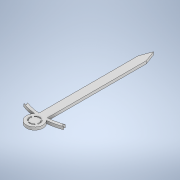
# Autodesk Inventor part: клинок
Saved by Autodesk Inventor 2022 (Build 260153000, 153)
## iProperties
Created: 2023-03-03
Part Number: клинок
Material: Типовые
Document SubType Name: Modeling
Designer: Папа
Density: 1 g/cm^3
Appearance: По умолчанию
Author: Папа
Autodesk Inventor part; units mm, degrees
ref_plane "YZ Plane" through (0, 0, 0) normal (1, 0, 0) x (0, 1, 0)
ref_plane "XZ Plane" through (0, 0, 0) normal (0, 1, 0) x (-1, 0, 0)
ref_plane "XY Plane" through (0, 0, 0) normal (0, 0, 1) x (1, 0, 0)
sketch "Эскиз1" plane through (0, 0, 0) normal (0, 1, 0) x (-1, 0, 0)
  arc A0 (15, -25.7496) -> (-15, -25.7496) centre (0, 0) ccw
  line L0 (0, 0) -> (0, -429.8) construction
  line L1 (15, -25.7496) -> (15, -388.5878)
  line L2 (15, -388.5878) -> (0, -429.8)
  line L3 (0, 0) -> (0, -29.8) construction
  circle A1 centre (0, 0) radius 17.5 construction
  circle A2 centre (0, -17.5) radius 1.6 construction
  line L4 (12.3744, -12.3744) -> (0, 0) construction
  arc A3 (-4.9434, -18.4492) -> (13.5057, -13.5057) centre (0, 0) ccw
  arc A4 (-4.1152, -15.3582) -> (11.243, -11.243) centre (0, 0) ccw
  arc A5 (-4.1152, -15.3582) -> (-4.9434, -18.4492) centre (-4.5293, -16.9037) ccw
  line L5 (0, 0) -> (-4.5293, -16.9037) construction
  arc A6 (13.5057, -13.5057) -> (11.243, -11.243) centre (12.3744, -12.3744) ccw
  arc A7 (18.4492, -4.9434) -> (13.5057, 13.5057) centre (0, 0) ccw
  circle A8 centre (17.5, 0) radius 1.6 construction
  arc A9 (15.3582, -4.1152) -> (11.243, 11.243) centre (0, 0) ccw
  arc A10 (15.3582, -4.1152) -> (18.4492, -4.9434) centre (16.9037, -4.5293) ccw
  arc A11 (13.5057, 13.5057) -> (11.243, 11.243) centre (12.3744, 12.3744) ccw
  arc A12 (4.9434, 18.4492) -> (-13.5057, 13.5057) centre (0, 0) ccw
  circle A13 centre (0, 17.5) radius 1.6 construction
  arc A14 (4.1152, 15.3582) -> (-11.243, 11.243) centre (0, 0) ccw
  arc A15 (4.1152, 15.3582) -> (4.9434, 18.4492) centre (4.5293, 16.9037) ccw
  arc A16 (-13.5057, 13.5057) -> (-11.243, 11.243) centre (-12.3744, 12.3744) ccw
  arc A17 (-18.4492, 4.9434) -> (-13.5057, -13.5057) centre (0, 0) ccw
  circle A18 centre (-17.5, 0) radius 1.6 construction
  arc A19 (-15.3582, 4.1152) -> (-11.243, -11.243) centre (0, 0) ccw
  arc A20 (-15.3582, 4.1152) -> (-18.4492, 4.9434) centre (-16.9037, 4.5293) ccw
  arc A21 (-13.5057, -13.5057) -> (-11.243, -11.243) centre (-12.3744, -12.3744) ccw
  line L6 (-15, -25.7496) -> (-15, -388.5878)
  line L7 (-15, -388.5878) -> (0, -429.8)
  circle A22 centre (0, -229.8) radius 200
  line L8 (0, -29.8) -> (0, -229.8) construction
  circle A23 centre (0, -229.8) radius 210
  line L9 (0, -229.8) -> (71.8242, -32.4645) construction
  line L10 (71.8242, -32.4645) -> (63.991, -34.9344)
  line L11 (63.991, -34.9344) -> (68.404, -41.8615)
  line L12 (-71.8242, -32.4645) -> (-63.991, -34.9344)
  line L13 (-63.991, -34.9344) -> (-68.404, -41.8615)
  point P0 (-15, -30.3633)
  point P1 (15, -30.3633)
  point P2 (21.2626, -20.8792)
  point P3 (-21.2626, -20.8792)
  point P4 (-71.8242, -32.4645)
  point P5 (-68.404, -41.8615)
  dimension "d0" = 59.6
  dimension "d1" = 400
  dimension "d2" = 20
  dimension "d3" = 15
  dimension "d4" = 35
  dimension "d5" = 3.2
  dimension "d6" = 45
  dimension "d7" = 15
  dimension "d8" = 3.2
  dimension "d11" = 360
  dimension "d14" = 29.8
  dimension "d15" = 200
  dimension "d17" = 20
  dimension "d18" = 75
  dimension "d19" = 10
  constraints: 39 point on circle, 28 end point, 23 centre point, 12 coincident, 5 symmetric about line, 3 point on line, 2 collinear, 2 equal radius, 2 vertical, 1 equal length, 1 tangent, 65 other
  measures "d0" diameter of A0
  measures "d1" distance of L0.end L3.end
  measures "d2" angle of L0 L2
  measures "d3" distance between parallel lines of L1 L0
  measures "d4" diameter of A1
  measures "d5" diameter of A2
  measures "d6" angle of L0 L4
  measures "d7" angle of L5 L3
  measures "d8" radial gap between concentric circles of A4 A3
  measures "d14" distance of point (0, 0) L3.end
  measures "d15" distance of L3.end L8.end
  measures "d17" angle of L9 L0
  measures "d18" angle of L11 L10
extrude "Выдавливание1" add sketch "Эскиз1" along normal blind 10 contours L1 A22 L6 A0 A23 | A0 A23 L10 L11 A22 L1 | A23 A0 | L1 L2 L7 L6 A22 | A0 L6 A22 L13 L12 A23
